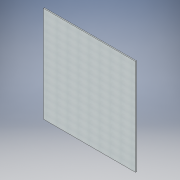
# Autodesk Inventor part: right_1_0
Saved by Autodesk Inventor 2019 (Build 230136000, 136)
## iProperties
Created: 2018-07-10
Part Number: right_1_0
Material: Generic
Document SubType Name: Modeling
Designer: User
Density: 1 g/cm^3
Appearance: Wood - Painted White
Author: User
Autodesk Inventor part; units mm, degrees
ref_plane "YZ Plane" through (0, 0, 0) normal (1, 0, 0) x (0, 1, 0)
ref_plane "XZ Plane" through (0, 0, 0) normal (0, 1, 0) x (-1, 0, 0)
ref_plane "XY Plane" through (0, 0, 0) normal (0, 0, 1) x (1, 0, 0)
sketch "Sketch1" plane through (0, 0, 0) normal (0, 0, 1) x (1, 0, 0)
  line L0 (-571.5, -596.9) -> (571.5, -596.9)
  line L1 (571.5, -596.9) -> (571.5, 596.9)
  line L2 (571.5, 596.9) -> (-571.5, 596.9)
  line L3 (-571.5, 596.9) -> (-571.5, -596.9)
  line L4 (-571.5, -596.9) -> (571.5, 596.9) construction
  line L5 (571.5, -596.9) -> (-571.5, 596.9) construction
  point P0 (0, 0)
  dimension "d0" = 1143
  dimension "d1" = 1193.8
  constraints: 12 end point, 2 midpoint, 2 parallel, 1 horizontal, 1 perpendicular
  measures "d0" distance of L1.end L2.end
  measures "d1" distance of L0.end L1.end
extrude "Extrusion1" add sketch "Sketch1" along normal blind 12.7
body "Solid1"
